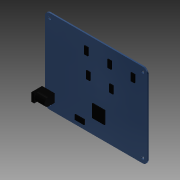
# Autodesk Inventor part: pcb
Saved by Autodesk Inventor 2013 (Build 170138000, 138)
## iProperties
Created: 2015-02-20
Part Number: pcb
Material: 一般
Document SubType Name: Modeling
Designer: Noa Izumi
Density: 1 g/cm^3
Author: Noa Izumi
Autodesk Inventor part; units mm, degrees
ref_plane "YZ Plane" through (0, 0, 0) normal (1, 0, 0) x (0, 1, 0)
ref_plane "XZ Plane" through (0, 0, 0) normal (0, 1, 0) x (-1, 0, 0)
ref_plane "XY Plane" through (0, 0, 0) normal (0, 0, 1) x (1, 0, 0)
sketch "草圖1" plane through (0, 0, 0) normal (0, 1, 0) x (-1, 0, 0)
  line L0 (0, 0) -> (110, 0)
  line L1 (110, 0) -> (110, 90)
  line L2 (110, 90) -> (0, 90)
  line L3 (0, 90) -> (0, 0)
  dimension "d0" = 110
  dimension "d1" = 90
  constraints: 8 end point, 2 parallel, 1 horizontal, 1 perpendicular
  measures "d0" distance of L0.start L0.end
  measures "d1" distance of L2.end L0.start
extrude "擠出1" add sketch "草圖1" along normal blind 1.4
fillet "圓角1" radius 5 4 edges at (0, 0.7, 90) (0, 0.7, 0) (-110, 0.7, 90) (-110, 0.7, 0)
sketch "草圖2" plane through (0, 0, 0) normal (0, -1, 0) x (1, 0, 0)
  line L0 (-5, 0) -> (-105, 0) projected
  line L1 (0, 85) -> (0, 5) projected
  line L2 (-105, 90) -> (-5, 90) projected
  line L3 (-110, 5) -> (-110, 85) projected
  point P0 (0, 0)
  point P1 (-105, 85)
  point P2 (-105, 5)
  point P3 (-5, 85)
  point P4 (-5, 5)
  dimension "d5" = 5
  dimension "d6" = 5
  dimension "d7" = 5
  dimension "d8" = 5
  measures "d5" distance from line of point (-105, 85) L2
  measures "d6" distance from line of point (-105, 85) L3
  measures "d7" distance from line of L1 point (-5, 85)
  measures "d8" distance from line of L0 point (-105, 5)
hole "孔1" at (-105, 0, 85) at (-105, 0, 5) at (-5, 0, 85) at (-5, 0, 5) direction (0, 1, 0) diameter 3 end through all
sketch "草圖3" plane through (0, 0, 0) normal (0, -1, 0) x (1, 0, 0)
  line L0 (-5, 0) -> (-105, 0) projected
  line L1 (-110, 5) -> (-110, 85) projected
  line L2 (-113, 18) -> (-99.5, 18)
  line L3 (-99.5, 18) -> (-99.5, 9)
  line L4 (-99.5, 9) -> (-113, 9)
  line L5 (-113, 9) -> (-113, 18)
  point P0 (0, 0)
  dimension "d16" = 9
  dimension "d17" = 9
  dimension "d18" = 13.5
  dimension "d19" = 3
  constraints: 8 end point, 2 parallel, 1 horizontal, 1 perpendicular
  measures "d16" distance between parallel lines of L0 L4
  measures "d17" distance of L4.end L2.start
  measures "d18" distance of L2.start L2.end
  measures "d19" distance between parallel lines of L1 L5
extrude "擠出2" add sketch "草圖3" along normal blind 11
sketch "草圖5" plane through (0, -11, 0) normal (0, -1, 0) x (1, 0, 0)
  line L0 (-113, 9) -> (-99.5, 9) projected
  line L1 (-113, 18) -> (-110, 18)
  line L2 (-110, 18) -> (-110, 9)
  line L3 (-110, 9) -> (-113, 9)
  line L4 (-113, 9) -> (-113, 18)
  point P0 (0, 0)
  dimension "d23" = 3
  constraints: 8 end point, 2 parallel, 1 horizontal, 1 perpendicular, 1 point on line
  measures "d23" distance of L1.start L1.end
extrude "擠出3" add sketch "草圖5" along normal blind 0.5
fillet "圓角2" radius 4.5 2 edges at (-104.75, -11, 18) (-104.75, -11, 9)
sketch "草圖7" plane through (-113, 0, 9) normal (-1, 0, 0) x (0, 0, 1)
  line L0 (9, -11.5) -> (0, -11.5) projected
  circle A0 centre (4.5, -7) radius 3
  circle A1 centre (4.5, -7) radius 0.75
  point P0 (-9, 0)
  dimension "d35" = 4.5
  dimension "d36" = 1.5
  dimension "d37" = 6
  constraints: 2 centre point, 1 coincident
  measures "d35" distance from line of L0 A1.centre
  measures "d36" diameter of A1
  measures "d37" diameter of A0
extrude "擠出4" cut sketch "草圖7" against normal blind 12
fillet "圓角3" radius 0.75 1 edges at (-113, -7, 12.75)
sketch "草圖8" plane through (0, 0, 0) normal (0, -1, 0) x (1, 0, 0)
  line L0 (-5, 0) -> (-105, 0) projected
  line L1 (0, 85) -> (0, 5) projected
  line L2 (-105, 90) -> (-5, 90) projected
  line L3 (-110, 18) -> (-110, 85) projected
  line L4 (-58.5, 29.5) -> (-45, 29.5)
  line L5 (-45, 29.5) -> (-45, 16)
  line L6 (-45, 16) -> (-58.5, 16)
  line L7 (-58.5, 16) -> (-58.5, 29.5)
  line L8 (-77, 10) -> (-67, 10)
  line L9 (-67, 10) -> (-67, 5)
  line L10 (-67, 5) -> (-77, 5)
  line L11 (-77, 5) -> (-77, 10)
  line L12 (-17, 79) -> (-13, 79)
  line L13 (-13, 79) -> (-13, 71)
  line L14 (-13, 71) -> (-17, 71)
  line L15 (-17, 71) -> (-17, 79)
  line L16 (-38, 79) -> (-42, 79)
  line L17 (-42, 79) -> (-42, 71)
  line L18 (-42, 71) -> (-38, 71)
  line L19 (-38, 71) -> (-38, 79)
  line L20 (-63, 71) -> (-67, 71)
  line L21 (-67, 71) -> (-67, 79)
  line L22 (-67, 79) -> (-63, 79)
  line L23 (-63, 79) -> (-63, 71)
  line L24 (-40, 57) -> (-36, 57)
  line L25 (-36, 57) -> (-36, 49)
  line L26 (-36, 49) -> (-40, 49)
  line L27 (-40, 49) -> (-40, 57)
  line L28 (-65, 57) -> (-61, 57)
  line L29 (-61, 57) -> (-61, 49)
  line L30 (-61, 49) -> (-65, 49)
  line L31 (-65, 49) -> (-65, 57)
  point P0 (0, 0)
  dimension "d41" = 13.5
  dimension "d43" = 13.5
  dimension "d44" = 51.5
  dimension "d45" = 16
  dimension "d46" = 10
  dimension "d47" = 5
  dimension "d48" = 33
  dimension "d49" = 5
  dimension "d50" = 4
  dimension "d51" = 8
  dimension "d52" = 13
  dimension "d53" = 11
  dimension "d54" = 4
  dimension "d55" = 4
  dimension "d56" = 21
  dimension "d57" = 21
  dimension "d58" = 4
  dimension "d59" = 8
  dimension "d60" = 2
  dimension "d61" = 14
  dimension "d62" = 4
  dimension "d63" = 21
  constraints: 56 end point, 14 parallel, 7 horizontal, 7 perpendicular
  measures "d41" distance of L4.start L4.end
  measures "d43" distance of L4.end L5.end
  measures "d44" distance between parallel lines of L3 L7
  measures "d45" distance between parallel lines of L0 L6
  measures "d46" distance of L8.start L8.end
  measures "d47" distance of L8.end L9.end
  measures "d48" distance between parallel lines of L11 L3
  measures "d49" distance between parallel lines of L0 L10
  measures "d50" distance of L13.end L14.end
  measures "d51" distance of L14.end L12.start
  measures "d52" distance between parallel lines of L1 L13
  measures "d53" distance between parallel lines of L12 L2
  measures "d54" distance of L20.start L20.end
  measures "d55" distance of L17.end L18.end
  measures "d56" distance between parallel lines of L15 L19
  measures "d57" distance between parallel lines of L23 L17
  measures "d58" distance of L24.start L24.end
  measures "d59" distance of L24.end L25.end
  measures "d60" distance between parallel lines of L25 L19
  measures "d61" distance between parallel lines of L24 L18
  measures "d62" distance of L29.end L30.end
  measures "d63" distance between parallel lines of L27 L29
extrude "擠出5" add sketch "草圖8" along normal blind 1
